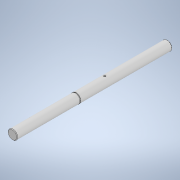
# Autodesk Inventor part: Håndtag
Saved by Autodesk Inventor 2022 (Build 260153000, 153)
## iProperties
Created: 2022-05-04
Part Number: Håndtag
Material: Generic
Document SubType Name: Modeling
Designer: Patrick
Density: 1 g/cm^3
Appearance: Default
Author: Patrick
Autodesk Inventor part; units mm, degrees
ref_plane "YZ Plane" through (0, 0, 0) normal (1, 0, 0) x (0, 1, 0)
ref_plane "XY Plane" through (0, 0, 0) normal (0, 0, 1) x (1, 0, 0)
sketch "Sketch1" plane through (0, 0, 0) normal (0, 1, 0) x (-1, 0, 0)
  line L0 (0, 0) -> (8, 0)
  line L1 (8, 0) -> (9, -1)
  line L2 (9, -1) -> (9, -121)
  line L3 (9, -121) -> (8.5, -121)
  line L4 (8.5, -121) -> (8.5, -122.5)
  line L5 (8.5, -122.5) -> (9, -122.5)
  line L6 (9, -297.5) -> (8.0002, -298.4998)
  line L7 (8.0002, -298.4998) -> (0, -298.4998)
  line L8 (0, -298.4998) -> (0, 0)
  line L9 (9, -122.5) -> (9, -297.5)
  dimension "d0" = 120
  dimension "d2" = 1.5
  dimension "d3" = 0.5
  dimension "d4" = 0.5
  dimension "d5" = 135
  dimension "d6" = 9
  dimension "d8" = 175
  dimension "d9" = 1.414
  dimension "d10" = 8
  constraints: 20 end point, 6 perpendicular, 1 parallel, 1 point on line, 1 vertical
  measures "d0" distance of L1.end L2.end
  measures "d2" distance of L3.end L4.end
  measures "d3" distance of L4.end L5.end
  measures "d4" distance of L2.end L3.end
  measures "d5" angle of L0 L1
  measures "d6" distance between parallel lines of L8 L2
  measures "d8" distance of L5.end L6.start
  measures "d9" distance of L6.start L6.end
  measures "d10" distance of L0.start L0.end
revolve "Shaft" add sketch "Sketch1" angle 360 about axis through (0, 0, -298.4998) along (0, 0, 1)
ref_plane "Hole for pin" through (0, 9, 0) normal (0, 1, 0) x (-1, 0, 0)
sketch "Sketch2" plane through (0, 9, 0) normal (0, 1, 0) x (-1, 0, 0)
  line L0 (-9, -122.5) -> (9, -122.5) projected
  line L1 (-9, -297.5) -> (9, -297.5) projected
  line L2 (-9, -122.5) -> (-9, -297.5) projected
  line L3 (9, -122.5) -> (9, -297.5) projected
  line L4 (9, -172.5) -> (-9, -172.5) construction
  circle A0 centre (0, -177.5) radius 1.75
  point P0 (0, 0)
  dimension "d13" = 50
  dimension "d14" = 3.5
  dimension "d15" = 5
  constraints: 2 end point, 2 point on line, 1 centre point, 1 perpendicular
  measures "d13" distance between parallel lines of L4 L0
  measures "d14" diameter of A0
  measures "d15" distance from line of L4 A0.centre
extrude "Pinhole" cut sketch "Sketch2" against normal through all contours A0
body "Solid1"
